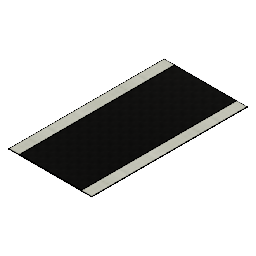
_Straight - Ruby.ad194a17-d179-4df3-b41d-e7b5ef9fd4d5 (Autodesk Fusion 360 design; units mm, degrees)
Autodesk Fusion 360 part; units mm, degrees
sketch "Sketch1" plane through (0, 0, 0) normal (0, 0, 1) x (1, 0, 0)
  line L0 (0, 0) -> (609.6, 0)
  line L1 (609.6, 0) -> (609.6, -1524)
  line L2 (609.6, -1524) -> (0, -1524)
  line L3 (0, -1524) -> (0, 0)
  line L4 (711.2, 101.6) -> (711.2, -1625.6)
  line L5 (711.2, -1625.6) -> (-101.6, -1625.6)
  line L6 (-101.6, -1625.6) -> (-101.6, 101.6)
  line L7 (-101.6, 101.6) -> (711.2, 101.6)
  line L8 (-101.6, 101.6) -> (711.2, 101.6)
  line L9 (711.2, 101.6) -> (711.2, 0)
  line L10 (711.2, 0) -> (-101.6, 0)
  line L11 (-101.6, 0) -> (-101.6, 101.6)
  line L12 (-101.6, -1625.6) -> (711.2, -1625.6)
  line L13 (711.2, -1625.6) -> (711.2, -1524)
  line L14 (711.2, -1524) -> (-101.6, -1524)
  line L15 (-101.6, -1524) -> (-101.6, -1625.6)
  dimension "d1" = 609.6
  dimension "d2" = 1524
  dimension "d3" = -101.6
  dimension "d4" = 101.6
  dimension "d5" = 101.6
  constraint horizontal L0
  constraint vertical L1
  constraint horizontal L2
  constraint vertical L3
  constraint coincident L0.start L3.end
  constraint horizontal L8
  constraint vertical L9
  constraint horizontal L10
  constraint vertical L11
  constraint horizontal L12
  constraint vertical L13
  constraint horizontal L14
  constraint vertical L15
  measures "d1" distance of L0.start L0.end
  measures "d2" distance of L0.start L2.end
  measures "d4" distance of L6.end L10.end
  measures "d5" distance of L5.end L14.end
extrude "Extrude1" add sketch "Sketch1" along normal blind 6.35 contours L0 L1 L2 L3 L10 L14 makes body 1
extrude "Extrude1'" add sketch "Sketch1" along normal blind 6.35 separate body contours L3 L6 L10 L14 | L1 L4 L10 L14 makes body 2 at (-67.7333, -1016, 0) makes body 3 at (643.4667, -1016, 0) in component "Straight"
copy_body "CutPasteBodies1" bodies 1 removing the originals makes body 4 in component "Straight"
component "Straight" placed x (1, 0, 0) y (0, 1, 0) z (0, 0, 1) at (0, 0, 0)
